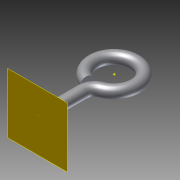
# Autodesk Inventor part: Eye_Pin_26Ga
Saved by Autodesk Inventor 2011 SP2 (Build 150309200, 309)
## iProperties
Created: 2011-04-01
Part Number: Eye_Pin_26Ga
Document SubType Name: Modeling
Designer: sungwook
Density: 1 g/cm^3
Author: sungwook
Autodesk Inventor part; units mm, degrees
ref_plane "YZ Plane" through (0, 0, 0) normal (1, 0, 0) x (0, 1, 0)
ref_plane "XY Plane" through (0, 0, 0) normal (0, 0, 1) x (1, 0, 0)
sketch "Block1" plane through (0, 0, 0) normal (0, 0, 1) x (1, 0, 0)
  line L0 (0, -0.4502) -> (0, -2)
  arc A0 (0.2899, 0.088) -> (-0.2, 0.0684) centre (0.0166, 0.7865) ccw
  arc A1 (0.2899, 0.088) -> (0, -0.3366) centre (0.456, -0.3366) ccw
  line L1 (0, -0.3366) -> (0, -0.519)
  point P0 (0.0505, -0.4167)
  point P1 (0.0166, -0.9635)
  dimension "d1" = 1.5
  measures "d1" diameter of A0
ref_plane "Work Plane1" through (0, -2, 0) normal (0, 1, 0) x (-1, 0, 0)
sketch "Sketch1" plane through (0, 0, 0) normal (0, 0, 1) x (1, 0, 0)
  line L0 (0, -0.4502) -> (0, -2)
  arc A0 (0.2899, 0.088) -> (-0.2, 0.0684) centre (0.0166, 0.7865) ccw
  arc A1 (0.2899, 0.088) -> (0, -0.3366) centre (0.456, -0.3366) ccw
  line L1 (0, -0.3366) -> (0, -0.519)
  point P0 (0, 0)
sketch "Sketch2" plane through (0, -2, 0) normal (0, 1, 0) x (-1, 0, 0)
  circle A0 centre (0, 0) radius 0.2032
  dimension "d4" = 0.4064
  constraints: 1 centre point, 1 coincident
  measures "d4" diameter of A0
sweep "Sweep1" [suppressed]
sweep "Sweep4" add profiles "Sketch2" path "Sketch1" path curves L0
sketch "Sketch4" plane through (0, -0.4502, 0) normal (0, 1, 0) x (1, 0, 0)
  circle A0 centre (0, 0) radius 0.2032 projected
sweep "Sweep5" add profiles "Sketch4" path "Sketch1" path curves L1 A1 A0
body "Solid1"
